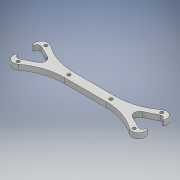
# Autodesk Inventor part: legFrame
Saved by Autodesk Inventor 2017 (Build 210142000, 142)
## iProperties
Created: 2016-08-27
Part Number: legFrame
Material: Generic
Document SubType Name: Modeling
Designer: Nic
Density: 1 g/cm^3
Appearance: Default
Author: Nic
Autodesk Inventor part; units mm, degrees
ref_plane "YZ Plane" through (0, 0, 0) normal (1, 0, 0) x (0, 1, 0)
ref_plane "XZ Plane" through (0, 0, 0) normal (0, 1, 0) x (-1, 0, 0)
ref_plane "XY Plane" through (0, 0, 0) normal (0, 0, 1) x (1, 0, 0)
sketch "Sketch1" plane through (0, 0, 0) normal (0, 0, 1) x (1, 0, 0)
  circle A0 centre (0, 0) radius 1.25
  circle A1 centre (-28.1025, 10.5) radius 1.25
  circle A2 centre (-28.1025, -10.5) radius 1.25
  line L0 (0, 0) -> (-28.1025, 0) construction
  line L1 (-28.1025, 10.5) -> (0, 0) construction
  line L2 (-28.1025, 0) -> (-28.1025, 10.5) construction
  circle A3 centre (0, 0) radius 2.5 construction
  circle A4 centre (-28.1025, 10.5) radius 2.5 construction
  circle A5 centre (-28.1025, -10.5) radius 2.5 construction
  line L3 (0, 0) -> (0, 7) construction
  line L4 (0, 3.5) -> (16, 3.5)
  arc A6 (-26.277, 12.2081) -> (0, 3.5) centre (0, 47.5) ccw
  line L5 (0, -3.5) -> (16, -3.5)
  line L6 (16, 0) -> (16, 5.5221) construction
  circle A7 centre (32, 0) radius 1.25
  circle A8 centre (60.1025, 10.5) radius 1.25
  circle A9 centre (60.1025, -10.5) radius 1.25
  line L7 (32, 0) -> (60.1025, 0) construction
  line L8 (60.1025, 10.5) -> (32, 0) construction
  line L9 (60.1025, 0) -> (60.1025, 10.5) construction
  circle A10 centre (32, 0) radius 2.5 construction
  circle A11 centre (60.1025, 10.5) radius 2.5 construction
  circle A12 centre (60.1025, -10.5) radius 2.5 construction
  line L10 (32, 0) -> (32, 7) construction
  line L11 (32, 3.5) -> (16, 3.5)
  line L12 (32, -3.5) -> (16, -3.5)
  arc A13 (-20.1367, -3.7476) -> (-20.1367, 3.7476) centre (-22, 0) ccw
  arc A14 (-26.277, 12.2081) -> (-33.7448, 6.3389) centre (-29.2155, 8.2614) ccw
  line L13 (-20.1367, 3.7476) -> (-29.2155, 8.2614)
  arc A15 (-29.2155, 8.2614) -> (-32.7919, 6.449) centre (-30.3285, 6.0228) ccw
  arc A16 (-33.7448, 6.3389) -> (-32.7919, 6.449) centre (-33.2846, 6.5343) ccw
  arc A17 (0, -3.5) -> (-26.277, -12.2081) centre (0, -47.5) ccw
  arc A18 (-33.7448, -6.3389) -> (-26.277, -12.2081) centre (-29.2155, -8.2614) ccw
  line L14 (-20.1367, -3.7476) -> (-29.2155, -8.2614)
  arc A19 (-32.7919, -6.449) -> (-29.2155, -8.2614) centre (-30.3285, -6.0228) ccw
  arc A20 (-32.7919, -6.449) -> (-33.7448, -6.3389) centre (-33.2846, -6.5343) ccw
  arc A21 (32, 3.5) -> (58.277, 12.2081) centre (32, 47.5) ccw
  arc A22 (52.1367, 3.7476) -> (52.1367, -3.7476) centre (54, 0) ccw
  arc A23 (65.7448, 6.3389) -> (58.277, 12.2081) centre (61.2155, 8.2614) ccw
  line L15 (52.1367, 3.7476) -> (61.2155, 8.2614)
  arc A24 (64.7919, 6.449) -> (61.2155, 8.2614) centre (62.3285, 6.0228) ccw
  arc A25 (64.7919, 6.449) -> (65.7448, 6.3389) centre (65.2846, 6.5343) ccw
  arc A26 (58.277, -12.2081) -> (32, -3.5) centre (32, -47.5) ccw
  arc A27 (58.277, -12.2081) -> (65.7448, -6.3389) centre (61.2155, -8.2614) ccw
  arc A28 (61.2155, -8.2614) -> (64.7919, -6.449) centre (62.3285, -6.0228) ccw
  line L16 (52.1367, -3.7476) -> (61.2155, -8.2614)
  arc A29 (65.7448, -6.3389) -> (64.7919, -6.449) centre (65.2846, -6.5343) ccw
  dimension "d0" = 2.5
  dimension "d1" = 10.5
  dimension "d2" = 30
  dimension "d3" = 5
  dimension "d22" = 3.5
  dimension "d27" = 16
  dimension "d32" = 0.5
  dimension "d36" = 22
  dimension "d37" = 2.5
  dimension "d38" = 0.5
  dimension "d45" = 88.205
  dimension "d47" = 44
  constraints: 40 point on circle, 40 symmetric about line, 34 end point, 30 centre point, 12 coincident, 9 tangent, 4 equal radius, 3 vertical, 2 horizontal, 2 point on line, 1 vertical alignment, 19 other
  measures "d0" diameter of A0
  measures "d1" distance of L0.end L1.start
  measures "d2" distance of L1.start L0.start
  measures "d3" diameter of A3
  measures "d22" distance from line of point (0, 0) L4
  measures "d27" distance from line of point (0, 0) L6
  measures "d32" radius of A16
  measures "d36" distance of point (0, 0) A13.centre
  measures "d37" radius of A15
  measures "d38" radius of A20
  measures "d45" distance of A9.centre A2.centre
  measures "d47" radius of A6
extrude "Extrusion1" add sketch "Sketch1" along normal blind 4
body "Solid1"
